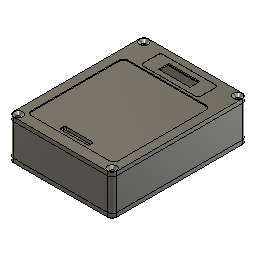
WiegandEmulator (Autodesk Fusion 360 design; units mm, degrees)
Autodesk Fusion 360 part; units mm, degrees
sketch "Sketch1" plane through (0, 0, 0) normal (0, 1, 0) x (1, 0, 0) in component "Core"
  line L0 (41.275, -53.975) -> (-41.275, -53.975)
  line L1 (-41.275, -53.975) -> (-41.275, 53.975)
  line L2 (-41.275, 53.975) -> (41.275, 53.975)
  line L3 (41.275, 53.975) -> (41.275, -53.975)
  line L4 (41.275, -53.975) -> (-41.275, 53.975) construction
  line L5 (-41.275, -53.975) -> (41.275, 53.975) construction
  dimension "d1" = 82.55
  dimension "d2" = 107.95
  constraint perpendicular L0 L1
  constraint parallel L0 L2
  constraint parallel L1 L3
  constraint horizontal L0
  constraint coincident L4 origin
  constraint coincident L5 origin
  measures "d1" distance of L1.end L2.end
  measures "d2" distance of L0.end L1.end
extrude "Extrude1" add sketch "Sketch1" along normal blind 25.4 makes body 1 in component "Core"
fillet "Fillet1" radius 3.81 4 edges at (41.275, 12.7, 53.975) (-41.275, 12.7, 53.975) (-41.275, 12.7, -53.975) (41.275, 12.7, -53.975) on bodies 1 in component "Core"
sketch "Sketch2" plane through (0, 25.4, 0) normal (0, 1, 0) x (-1, 0, 0) in component "Core"
  line L0 (-37.465, -53.975) -> (37.465, -53.975)
  line L1 (41.275, -50.165) -> (41.275, 50.165)
  line L2 (37.465, 53.975) -> (-37.465, 53.975)
  line L3 (-41.275, 50.165) -> (-41.275, -50.165)
  arc A0 (-41.275, -50.165) -> (-37.465, -53.975) centre (-37.465, -50.165) ccw
  arc A1 (37.465, -53.975) -> (41.275, -50.165) centre (37.465, -50.165) ccw
  arc A2 (41.275, 50.165) -> (37.465, 53.975) centre (37.465, 50.165) ccw
  arc A3 (-37.465, 53.975) -> (-41.275, 50.165) centre (-37.465, 50.165) ccw
  circle A4 centre (-37.465, 50.165) radius 1.8542
  circle A5 centre (37.465, 50.165) radius 1.8542
  circle A6 centre (37.465, -50.165) radius 1.8542
  circle A7 centre (-37.465, -50.165) radius 1.8542
  line L4 (38.735, -58.42) -> (38.735, 58.42) construction
  line L5 (-38.735, -46.5729) -> (-38.735, 46.5729)
  line L6 (-33.8729, 51.435) -> (33.8729, 51.435)
  line L7 (38.735, 46.5729) -> (38.735, -46.5729)
  arc A8 (41.0571, -51.435) -> (41.275, -50.165) centre (37.465, -50.165) ccw
  arc A9 (38.735, -46.5729) -> (33.8729, -51.435) centre (37.465, -50.165) ccw
  line L8 (33.8729, -51.435) -> (-33.8729, -51.435)
  line L9 (-38.735, -51.435) -> (-38.735, -51.516) construction
  arc A10 (-33.8729, -51.435) -> (-38.735, -46.5729) centre (-37.465, -50.165) ccw
  line L10 (-43.18, -51.435) -> (-41.0571, -51.435) construction
  line L11 (-38.816, -51.435) -> (-38.735, -51.435) construction
  line L12 (-33.8729, -51.435) -> (43.18, -51.435) construction
  arc A11 (33.8729, 51.435) -> (38.735, 46.5729) centre (37.465, 50.165) ccw
  arc A12 (-38.735, 46.5729) -> (-33.8729, 51.435) centre (-37.465, 50.165) ccw
  line L13 (-38.735, 51.516) -> (-38.735, 51.435) construction
  line L14 (-38.735, 46.5729) -> (-38.735, -46.5729) construction
  line L15 (43.18, 51.435) -> (-33.8729, 51.435) construction
  line L16 (-38.735, 51.435) -> (-38.816, 51.435) construction
  dimension "d10" = 3.7084
  dimension "d11" = 3.7084
  dimension "d12" = 3.7084
  dimension "d13" = 3.7084
  dimension "d14" = 2.54
  dimension "d15" = 2.54
  dimension "d16" = 2.54
  dimension "d17" = 2.54
  dimension "d18" = 3.81
  dimension "d19" = 3.81
  dimension "d21" = 3.81
  dimension "d22" = 3.81
  constraint concentric A3 A4
  constraint concentric A2 A5
  constraint concentric A1 A6
  constraint concentric A0 A7
  constraint perpendicular L0 L4
  constraint perpendicular L4 L15
  constraint perpendicular L13 L15
  constraint perpendicular L1 L10
  constraint concentric A1 A9
  constraint concentric A0 A10
  constraint coincident L5.end L13
  constraint coincident L6.end L15
  constraint coincident L4 L7.start
  constraint coincident L4 L7.end
  constraint coincident A8.start L10
  constraint concentric A8 A9
  constraint coincident A9.end L10
  constraint coincident L8.end L10
  constraint coincident A7 L9.end
  constraint coincident L9.start L10
  constraint collinear L9 L13
  constraint coincident A0 L10.end
  constraint coincident A7 L11.start
  constraint collinear L10 L11
  constraint collinear L11 L12
  constraint coincident A4 L13.start
  constraint collinear L13 L14
  constraint coincident L13.end L15
  constraint collinear L15 L16
  constraint coincident A4 L16.end
  constraint horizontal A2.centre A3.centre
  constraint vertical A1.centre A2.centre
  constraint vertical A0.centre A3.centre
  measures "d10" diameter of A4
  measures "d11" diameter of A5
  measures "d12" diameter of A6
  measures "d13" diameter of A7
  measures "d14" distance of L0 L10
  measures "d15" distance of L3 L13
  measures "d16" distance of L2 L15
  measures "d17" distance of L1 L4
  measures "d18" radius of A10
  measures "d19" radius of A9
  measures "d21" radius of A11
  measures "d22" radius of A12
extrude "Extrude2" cut sketch "Sketch2" against normal through all contours A4 | A5 | A6 | A7 | L5 L6 L7 A9 L8 A10 A11 A12 bodies 1 in component "Core"
sketch "Sketch1 (2)" plane through (0, 25.4, 0) normal (0, 1, 0) x (-1, 0, 0) in component "TopLid"
  circle A0 centre (-37.465, 50.165) radius 1.8542
  circle A1 centre (37.465, 50.165) radius 1.8542
  circle A2 centre (37.465, -50.165) radius 1.8542
  arc A3 (33.8729, 51.435) -> (38.735, 46.5729) centre (37.465, 50.165) ccw
  line L0 (38.735, 46.5729) -> (38.735, -46.5729)
  arc A4 (38.735, -46.5729) -> (33.8729, -51.435) centre (37.465, -50.165) ccw
  line L1 (33.8729, -51.435) -> (-33.8729, -51.435)
  arc A5 (-33.8729, -51.435) -> (-38.735, -46.5729) centre (-37.465, -50.165) ccw
  line L2 (-38.735, -46.5729) -> (-38.735, 46.5729)
  arc A6 (-38.735, 46.5729) -> (-33.8729, 51.435) centre (-37.465, 50.165) ccw
  line L3 (-33.8729, 51.435) -> (33.8729, 51.435)
  circle A7 centre (-37.465, -50.165) radius 1.8542
  arc A8 (-41.275, -50.165) -> (-37.465, -53.975) centre (-37.465, -50.165) ccw
  line L4 (-37.465, -53.975) -> (37.465, -53.975)
  arc A9 (37.465, -53.975) -> (41.275, -50.165) centre (37.465, -50.165) ccw
  line L5 (41.275, -50.165) -> (41.275, 50.165)
  arc A10 (41.275, 50.165) -> (37.465, 53.975) centre (37.465, 50.165) ccw
  line L6 (37.465, 53.975) -> (-37.465, 53.975)
  arc A11 (-37.465, 53.975) -> (-41.275, 50.165) centre (-37.465, 50.165) ccw
  line L7 (-41.275, 50.165) -> (-41.275, -50.165)
  line L8 (41.275, -50.165) -> (41.275, 50.165)
  arc A12 (41.275, 50.165) -> (37.465, 53.975) centre (37.465, 50.165) ccw
  line L9 (37.465, 53.975) -> (-37.465, 53.975)
  arc A13 (-37.465, 53.975) -> (-41.275, 50.165) centre (-37.465, 50.165) ccw
  line L10 (-41.275, 50.165) -> (-41.275, -50.165)
  arc A14 (-41.275, -50.165) -> (-37.465, -53.975) centre (-37.465, -50.165) ccw
  line L11 (-37.465, -53.975) -> (37.465, -53.975)
  arc A15 (37.465, -53.975) -> (41.275, -50.165) centre (37.465, -50.165) ccw
  circle A16 centre (37.465, -50.165) radius 1.8542
  circle A17 centre (37.465, 50.165) radius 1.8542
  circle A18 centre (-37.465, 50.165) radius 1.8542
  circle A19 centre (-37.465, -50.165) radius 1.8542
  circle A20 centre (-37.465, 50.165) radius 1.524
  circle A21 centre (37.465, 50.165) radius 1.524
  circle A22 centre (37.465, -50.165) radius 1.524
  circle A23 centre (-37.465, -50.165) radius 1.524
  dimension "d26" = 3.048
  dimension "d27" = 3.048
  dimension "d28" = 3.048
  dimension "d29" = 3.048
  constraint concentric A18 A20
  constraint concentric A12 A21
  constraint concentric A16 A22
  constraint concentric A14 A23
  measures "d26" diameter of A20
  measures "d27" diameter of A21
  measures "d28" diameter of A22
  measures "d29" diameter of A23
extrude "Extrude1'" add sketch "Sketch1 (2)" along normal blind 3.175 separate body contours A0 A18 | A1 A17 | A2 A16 | A3 L0 A4 L1 A5 L2 A6 L3 | A7 A19 | A8 L4 A9 L5 A10 L6 A11 L7 L8 A12 L9 A13 L10 A14 L11 A15 | A20 | A21 | A22 | A23 makes body 2 in component "TopLid"
extrude "Extrude2'" cut sketch "Sketch1 (2)" along normal through all contours A20 | A21 | A22 | A23 bodies 2 in component "TopLid"
sketch "Sketch2 (2)" plane through (0, 28.575, 0) normal (0, 1, 0) x (-1, 0, 0) in component "TopLid"
  circle A0 centre (-37.465, 50.165) radius 1.524
  circle A1 centre (-37.465, -50.165) radius 1.524
  circle A2 centre (37.465, 50.165) radius 1.524
  circle A3 centre (37.465, -50.165) radius 1.524
  arc A4 (37.465, -53.975) -> (41.275, -50.165) centre (37.465, -50.165) ccw
  line L0 (41.275, -50.165) -> (41.275, 50.165)
  arc A5 (41.275, 50.165) -> (37.465, 53.975) centre (37.465, 50.165) ccw
  line L1 (37.465, 53.975) -> (-37.465, 53.975)
  arc A6 (-37.465, 53.975) -> (-41.275, 50.165) centre (-37.465, 50.165) ccw
  line L2 (-41.275, 50.165) -> (-41.275, -50.165)
  arc A7 (-41.275, -50.165) -> (-37.465, -53.975) centre (-37.465, -50.165) ccw
  line L3 (-37.465, -53.975) -> (37.465, -53.975)
  line L4 (31.171, 45.975) -> (-31.171, 45.975)
  line L5 (-34.671, 42.475) -> (-34.671, -27.525)
  line L6 (-31.171, -31.025) -> (31.171, -31.025)
  line L7 (34.671, -27.525) -> (34.671, 42.475)
  arc A8 (34.671, 42.475) -> (31.171, 45.975) centre (31.171, 42.475) ccw
  arc A9 (-34.671, -27.525) -> (-31.171, -31.025) centre (-31.171, -27.525) ccw
  line L8 (34.671, -31.025) -> (-34.671, 45.975) construction
  arc A10 (31.171, -31.025) -> (34.671, -27.525) centre (31.171, -27.525) ccw
  arc A11 (-31.171, 45.975) -> (-34.671, 42.475) centre (-31.171, 42.475) ccw
  line L9 (-21, -49.025) -> (21, -49.025)
  line L10 (23, -47.025) -> (23, -35.025)
  line L11 (21, -33.025) -> (-21, -33.025)
  line L12 (-23, -35.025) -> (-23, -47.025)
  line L13 (-23, -49.025) -> (23, -33.025) construction
  line L14 (23, -49.025) -> (-23, -33.025) construction
  arc A12 (21, -49.025) -> (23, -47.025) centre (21, -47.025) ccw
  arc A13 (23, -35.025) -> (21, -33.025) centre (21, -35.025) ccw
  arc A14 (-21, -33.025) -> (-23, -35.025) centre (-21, -35.025) ccw
  arc A15 (-23, -47.025) -> (-21, -49.025) centre (-21, -47.025) ccw
  point P0 (34.671, 45.975)
  point P1 (0, -41.025)
  dimension "d31" = 69.342
  dimension "d32" = 77
  dimension "d33" = 34.671
  dimension "d34" = 8
  dimension "d35" = 3.5
  dimension "d36" = 3.5
  dimension "d37" = 3.5
  dimension "d38" = 3.5
  dimension "d50" = 46
  dimension "d51" = 16
  dimension "d52" = 10
  dimension "d53" = 11.671
  dimension "d54" = 2
  dimension "d55" = 2
  dimension "d56" = 2
  dimension "d57" = 2
  constraint horizontal L4
  constraint vertical L5
  constraint horizontal L6
  constraint vertical L7
  constraint coincident P0 L7
  constraint coincident P0 L4
  constraint tangent L7 A8
  constraint tangent L4 A8
  constraint tangent L6 A9
  constraint tangent L5 A9
  constraint coincident L8.start L6
  constraint coincident L8.start L7
  constraint tangent L6 A10
  constraint tangent L7 A10
  constraint coincident L8.end L4
  constraint coincident L8.end L5
  constraint tangent L4 A11
  constraint tangent L5 A11
  constraint perpendicular L9 L10
  constraint parallel L9 L11
  constraint parallel L10 L12
  constraint horizontal L9
  constraint coincident L13 P1
  constraint coincident L14 P1
  constraint coincident L14.start L9
  constraint coincident L14.start L10
  constraint tangent L9 A12
  constraint tangent L10 A12
  constraint coincident L13.end L10
  constraint coincident L13.end L11
  constraint tangent L10 A13
  constraint tangent L11 A13
  constraint coincident L14.end L12
  constraint coincident L14.end L11
  constraint tangent L12 A14
  constraint tangent L11 A14
  constraint coincident L13.start L9
  constraint coincident L13.start L12
  constraint tangent L9 A15
  constraint tangent L12 A15
  measures "d31" distance of P0 L8.end
  measures "d32" distance of P0 L8.start
  measures "d33" distance of origin L7
  measures "d34" distance of L1 L4
  measures "d35" radius of A8
  measures "d36" radius of A9
  measures "d37" radius of A10
  measures "d38" radius of A11
  measures "d50" distance of L13.end L14.end
  measures "d51" distance of L14.start L13.end
  measures "d52" distance of L6 P1
  measures "d53" distance of L7 L10
  measures "d54" radius of A12
  measures "d55" radius of A13
  measures "d56" radius of A14
  measures "d57" radius of A15
extrude "Extrude3" cut sketch "Sketch2 (2)" against normal blind 0.75 contours L4 L5 L6 L7 A8 A9 A10 A11 bodies 2 in component "TopLid"
sketch "Sketch3" plane through (0, 27.825, 0) normal (0, 1, 0) x (-1, 0, 0) in component "TopLid"
  arc A0 (-31.171, 45.975) -> (-34.671, 42.475) centre (-31.171, 42.475) ccw
  line L0 (-34.671, 42.475) -> (-34.671, -27.525)
  arc A1 (-34.671, -27.525) -> (-31.171, -31.025) centre (-31.171, -27.525) ccw
  line L1 (-31.171, -31.025) -> (31.171, -31.025)
  arc A2 (31.171, -31.025) -> (34.671, -27.525) centre (31.171, -27.525) ccw
  line L2 (34.671, -27.525) -> (34.671, 42.475)
  arc A3 (34.671, 42.475) -> (31.171, 45.975) centre (31.171, 42.475) ccw
  line L3 (31.171, 45.975) -> (-31.171, 45.975)
  line L4 (10.5, 42.975) -> (-10.5, 42.975)
  line L5 (-11.5, 41.975) -> (-11.5, 39.975)
  line L6 (-10.5, 38.975) -> (10.5, 38.975)
  line L7 (11.5, 39.975) -> (11.5, 41.975)
  arc A4 (11.5, 41.975) -> (10.5, 42.975) centre (10.5, 41.975) ccw
  arc A5 (10.5, 38.975) -> (11.5, 39.975) centre (10.5, 39.975) ccw
  arc A6 (-10.5, 42.975) -> (-11.5, 41.975) centre (-10.5, 41.975) ccw
  arc A7 (-11.5, 39.975) -> (-10.5, 38.975) centre (-10.5, 39.975) ccw
  point P0 (11.5, 42.975)
  point P1 (-11.5, 42.975)
  point P2 (11.5, 38.975)
  dimension "d41" = 23
  dimension "d42" = 4
  dimension "d43" = 11.5
  dimension "d44" = 7
  dimension "d45" = 1
  dimension "d46" = 1
  dimension "d47" = 1
  dimension "d48" = 1
  constraint horizontal L4
  constraint vertical L5
  constraint horizontal L6
  constraint vertical L7
  constraint coincident P0 L4
  constraint coincident P0 L7
  constraint tangent L4 A4
  constraint tangent L7 A4
  constraint coincident P2 L6
  constraint coincident P2 L7
  constraint tangent L6 A5
  constraint tangent L7 A5
  constraint coincident P1 L4
  constraint coincident P1 L5
  constraint tangent L4 A6
  constraint tangent L5 A6
  constraint tangent L5 A7
  constraint tangent L6 A7
  measures "d41" distance of P0 P1
  measures "d42" distance of P0 P2
  measures "d43" distance of origin L5
  measures "d44" distance of L3 L6
  measures "d45" radius of A4
  measures "d46" radius of A5
  measures "d47" radius of A6
  measures "d48" radius of A7
extrude "Extrude4" cut sketch "Sketch3" against normal through all contours L4 L5 L6 L7 A4 A5 A6 A7 bodies 2 in component "TopLid"
extrude "Extrude5" cut sketch "Sketch2 (2)" against normal through all contours L9 L10 L11 L12 A12 A13 A14 A15 bodies 2 in component "TopLid"
chamfer "Chamfer2" distance 2 angle 45 4 edges at (-36.0441, 28.575, 50.7161) (38.8859, 28.575, 50.7161) (-36.0441, 28.575, -49.6139) (38.8859, 28.575, -49.6139) on bodies 2 in component "TopLid"
sketch "Sketch1 (3)" plane through (0, 0, 0) normal (0, -1, 0) x (1, 0, 0) in component "BottomLid"
  circle A0 centre (37.465, 50.165) radius 1.8542
  circle A1 centre (-37.465, 50.165) radius 1.8542
  circle A2 centre (-37.465, -50.165) radius 1.8542
  arc A3 (-38.735, 46.5729) -> (-33.8729, 51.435) centre (-37.465, 50.165) ccw
  line L0 (-33.8729, 51.435) -> (33.8729, 51.435)
  arc A4 (33.8729, 51.435) -> (38.735, 46.5729) centre (37.465, 50.165) ccw
  line L1 (38.735, 46.5729) -> (38.735, -46.5729)
  arc A5 (38.735, -46.5729) -> (33.8729, -51.435) centre (37.465, -50.165) ccw
  line L2 (33.8729, -51.435) -> (-33.8729, -51.435)
  arc A6 (-33.8729, -51.435) -> (-38.735, -46.5729) centre (-37.465, -50.165) ccw
  line L3 (-38.735, -46.5729) -> (-38.735, 46.5729)
  circle A7 centre (37.465, -50.165) radius 1.8542
  arc A8 (37.465, -53.975) -> (41.275, -50.165) centre (37.465, -50.165) ccw
  line L4 (41.275, -50.165) -> (41.275, 50.165)
  arc A9 (41.275, 50.165) -> (37.465, 53.975) centre (37.465, 50.165) ccw
  line L5 (37.465, 53.975) -> (-37.465, 53.975)
  arc A10 (-37.465, 53.975) -> (-41.275, 50.165) centre (-37.465, 50.165) ccw
  line L6 (-41.275, 50.165) -> (-41.275, -50.165)
  arc A11 (-41.275, -50.165) -> (-37.465, -53.975) centre (-37.465, -50.165) ccw
  line L7 (-37.465, -53.975) -> (37.465, -53.975)
  line L8 (-41.275, 50.165) -> (-41.275, -50.165)
  arc A12 (-37.465, 53.975) -> (-41.275, 50.165) centre (-37.465, 50.165) ccw
  line L9 (37.465, 53.975) -> (-37.465, 53.975)
  arc A13 (41.275, 50.165) -> (37.465, 53.975) centre (37.465, 50.165) ccw
  line L10 (41.275, -50.165) -> (41.275, 50.165)
  arc A14 (37.465, -53.975) -> (41.275, -50.165) centre (37.465, -50.165) ccw
  line L11 (-37.465, -53.975) -> (37.465, -53.975)
  arc A15 (-41.275, -50.165) -> (-37.465, -53.975) centre (-37.465, -50.165) ccw
  circle A16 centre (-37.465, 50.165) radius 1.8542
  circle A17 centre (37.465, 50.165) radius 1.8542
  circle A18 centre (37.465, -50.165) radius 1.8542
  circle A19 centre (-37.465, -50.165) radius 1.8542
extrude "Extrude1''" add sketch "Sketch1 (3)" along normal blind 3.175 separate body contours A3 L0 A4 L1 A5 L2 A6 L3 | A8 L4 A9 L5 A10 L6 A11 L7 L8 A12 L9 A13 L10 A14 L11 A15 makes body 3 in component "BottomLid"
chamfer "Chamfer1" distance 1.75 angle 45 4 edges at (35.7363, -3.175, 50.8355) (-39.1937, -3.175, 50.8355) (-39.1937, -3.175, -49.4945) (35.7363, -3.175, -49.4945) on bodies 3 in component "BottomLid"
sketch "Sketch2 (3)" plane through (0, 0, 0) normal (0, 1, 0) x (-1, 0, 0) in component "BottomLid"
  circle A0 centre (-37.465, 50.165) radius 1.8542
  circle A1 centre (-37.465, -50.165) radius 1.8542
  circle A2 centre (37.465, -50.165) radius 1.8542
  circle A3 centre (37.465, 50.165) radius 1.8542
  arc A4 (37.465, -53.975) -> (41.275, -50.165) centre (37.465, -50.165) ccw
  line L0 (41.275, -50.165) -> (41.275, 50.165)
  arc A5 (41.275, 50.165) -> (37.465, 53.975) centre (37.465, 50.165) ccw
  line L1 (37.465, 53.975) -> (-37.465, 53.975)
  arc A6 (-37.465, 53.975) -> (-41.275, 50.165) centre (-37.465, 50.165) ccw
  line L2 (-41.275, 50.165) -> (-41.275, -50.165)
  arc A7 (-41.275, -50.165) -> (-37.465, -53.975) centre (-37.465, -50.165) ccw
  line L3 (-37.465, -53.975) -> (37.465, -53.975)
  circle A8 centre (0, -38.975) radius 6.1
  circle A9 centre (0, 38.975) radius 6.1
  dimension "d64" = 12.2
  dimension "d65" = 12.2
  dimension "d66" = 15
  dimension "d67" = 15
  dimension "d68" = 41.275
  constraint vertical A8.centre A9.centre
  measures "d64" diameter of A8
  measures "d65" diameter of A9
  measures "d66" distance of L1 A9.centre
  measures "d67" distance of L3 A8.centre
  measures "d68" distance of L2 A8.centre
extrude "Extrude2''" cut sketch "Sketch2 (3)" against normal blind 2.54 contours A8 | A9 bodies 3 in component "BottomLid"
fillet "Fillet1'" radius 0.5 2 edges at (5.6872, 0, 41.1809) (5.6872, 0, -36.7691) on bodies 3 in component "BottomLid"
ref_plane "WorkPlane1" through (0, 25.4, 0) normal (0, -1, 0) x (1, 0, 0) in component "DisplayInsert"
sketch "Sketch1 (4)" plane through (0, 25.4, 0) normal (0, -1, 0) x (1, 0, 0) in component "DisplayInsert"
  line L0 (-21, -49.025) -> (21, -49.025)
  arc A0 (21, -49.025) -> (23, -47.025) centre (21, -47.025) ccw
  line L1 (23, -47.025) -> (23, -35.025)
  arc A1 (23, -35.025) -> (21, -33.025) centre (21, -35.025) ccw
  line L2 (21, -33.025) -> (-21, -33.025)
  arc A2 (-21, -33.025) -> (-23, -35.025) centre (-21, -35.025) ccw
  line L3 (-23, -35.025) -> (-23, -47.025)
  arc A3 (-23, -47.025) -> (-21, -49.025) centre (-21, -47.025) ccw
  line L4 (23.5, -47.025) -> (23.5, -35.025)
  arc A4 (23.5, -35.025) -> (21, -32.525) centre (21, -35.025) ccw
  line L5 (21, -32.525) -> (-21, -32.525)
  arc A5 (-21, -32.525) -> (-23.5, -35.025) centre (-21, -35.025) ccw
  line L6 (-23.5, -35.025) -> (-23.5, -47.025)
  arc A6 (-23.5, -47.025) -> (-21, -49.525) centre (-21, -47.025) ccw
  line L7 (-21, -49.525) -> (21, -49.525)
  arc A7 (21, -49.525) -> (23.5, -47.025) centre (21, -47.025) ccw
  line L8 (22.9, -47.025) -> (22.9, -35.025)
  arc A8 (22.9, -35.025) -> (21, -33.125) centre (21, -35.025) ccw
  line L9 (21, -33.125) -> (-21, -33.125)
  arc A9 (-21, -33.125) -> (-22.9, -35.025) centre (-21, -35.025) ccw
  line L10 (-22.9, -35.025) -> (-22.9, -47.025)
  arc A10 (-22.9, -47.025) -> (-21, -48.925) centre (-21, -47.025) ccw
  line L11 (-21, -48.925) -> (21, -48.925)
  arc A11 (21, -48.925) -> (22.9, -47.025) centre (21, -47.025) ccw
  dimension "d73" = 0.5
  dimension "d89" = -0.1
extrude "Extrude1'''" add sketch "Sketch1 (4)" against normal blind 3.175 separate body contours L8 A8 L9 A9 L10 A10 L11 A11 makes body 4 in component "DisplayInsert"
extrude "Extrude2'''" add sketch "Sketch1 (4)" along normal blind 1 contours L0 A0 L1 A1 L2 A2 L3 A3 | L4 A4 L5 A5 L6 A6 L7 A7 | L8 A8 L9 A9 L10 A10 L11 A11 bodies 4 in component "DisplayInsert"
sketch "Sketch2 (4)" plane through (0, 28.575, 0) normal (0, 1, 0) x (-1, 0, 0) in component "DisplayInsert"
  line L0 (-12.5, -37.025) -> (12.5, -37.025)
  line L1 (12.5, -37.025) -> (12.5, -45.025)
  line L2 (12.5, -45.025) -> (-12.5, -45.025)
  line L3 (-12.5, -45.025) -> (-12.5, -37.025)
  line L4 (-12.5, -37.025) -> (12.5, -45.025) construction
  line L5 (12.5, -37.025) -> (-12.5, -45.025) construction
  arc A0 (-22.9, -47.025) -> (-21, -48.925) centre (-21, -47.025) ccw
  line L6 (-21, -48.925) -> (21, -48.925)
  arc A1 (21, -48.925) -> (22.9, -47.025) centre (21, -47.025) ccw
  line L7 (22.9, -47.025) -> (22.9, -35.025)
  arc A2 (22.9, -35.025) -> (21, -33.125) centre (21, -35.025) ccw
  line L8 (21, -33.125) -> (-21, -33.125)
  arc A3 (-21, -33.125) -> (-22.9, -35.025) centre (-21, -35.025) ccw
  line L9 (-22.9, -35.025) -> (-22.9, -47.025)
  point P0 (0, -41.025)
  dimension "d78" = 25
  dimension "d79" = 8
  dimension "d90" = 10.4
  dimension "d91" = 3.9
  constraint perpendicular L0 L1
  constraint parallel L0 L2
  constraint parallel L1 L3
  constraint horizontal L0
  constraint coincident L4 P0
  constraint coincident L5 P0
  measures "d78" distance of L1.end L2.end
  measures "d79" distance of L0.end L1.end
  measures "d90" distance of L3 L9
  measures "d91" distance of L2 L6
extrude "Extrude3'" cut sketch "Sketch2 (4)" against normal through all contours L0 L1 L2 L3 bodies 4 in component "DisplayInsert"
sketch "Sketch3 (2)" plane through (0, 24.4, 0) normal (0, -1, 0) x (1, 0, 0) in component "DisplayInsert"
  line L0 (12.5, -37.025) -> (12.5, -45.025)
  line L1 (12.5, -45.025) -> (-12.5, -45.025)
  line L2 (-12.5, -45.025) -> (-12.5, -37.025)
  line L3 (-12.5, -37.025) -> (12.5, -37.025)
  arc A0 (21, -49.525) -> (23.5, -47.025) centre (21, -47.025) ccw
  line L4 (23.5, -47.025) -> (23.5, -35.025)
  arc A1 (23.5, -35.025) -> (21, -32.525) centre (21, -35.025) ccw
  line L5 (21, -32.525) -> (-21, -32.525)
  arc A2 (-21, -32.525) -> (-23.5, -35.025) centre (-21, -35.025) ccw
  line L6 (-23.5, -35.025) -> (-23.5, -47.025)
  arc A3 (-23.5, -47.025) -> (-21, -49.525) centre (-21, -47.025) ccw
  line L7 (-21, -49.525) -> (21, -49.525)
  line L8 (18.75, -47.525) -> (-19.75, -47.525)
  line L9 (-19.75, -47.525) -> (-19.75, -34.525)
  line L10 (-19.75, -34.525) -> (18.75, -34.525)
  line L11 (18.75, -34.525) -> (18.75, -47.525)
  line L12 (18.75, -47.525) -> (-19.75, -34.525) construction
  line L13 (-19.75, -47.525) -> (18.75, -34.525) construction
  point P0 (-0.5, -41.025)
  dimension "d83" = 38.5
  dimension "d84" = 13
  dimension "d85" = 7.25
  dimension "d86" = 2.5
  constraint perpendicular L8 L9
  constraint parallel L8 L10
  constraint parallel L9 L11
  constraint horizontal L8
  constraint coincident L12 P0
  constraint coincident L13 P0
  measures "d83" distance of L9.end L10.end
  measures "d84" distance of L8.end L9.end
  measures "d85" distance of L2 L9
  measures "d86" distance of L3 L10
extrude "Extrude4'" cut sketch "Sketch3 (2)" against normal blind 3.2 contours L8 L9 L10 L11 bodies 4 in component "DisplayInsert"
sketch "Sketch1 (5)" plane through (0, 25.4, 0) normal (0, -1, 0) x (1, 0, 0) in component "ArduinoHolder"
  line L0 (-21, -33.025) -> (21, -33.025)
  arc A0 (23, -35.025) -> (21, -33.025) centre (21, -35.025) ccw
  line L1 (23, -35.025) -> (23, -47.025)
  arc A1 (21, -49.025) -> (23, -47.025) centre (21, -47.025) ccw
  line L2 (21, -49.025) -> (-21, -49.025)
  arc A2 (-23, -47.025) -> (-21, -49.025) centre (-21, -47.025) ccw
  line L3 (-23, -47.025) -> (-23, -35.025)
  arc A3 (-21, -33.025) -> (-23, -35.025) centre (-21, -35.025) ccw
  line L4 (-10.5, 42.975) -> (10.5, 42.975)
  arc A4 (11.5, 41.975) -> (10.5, 42.975) centre (10.5, 41.975) ccw
  line L5 (11.5, 41.975) -> (11.5, 39.975)
  arc A5 (10.5, 38.975) -> (11.5, 39.975) centre (10.5, 39.975) ccw
  line L6 (10.5, 38.975) -> (-10.5, 38.975)
  arc A6 (-11.5, 39.975) -> (-10.5, 38.975) centre (-10.5, 39.975) ccw
  line L7 (-11.5, 39.975) -> (-11.5, 41.975)
  arc A7 (-10.5, 42.975) -> (-11.5, 41.975) centre (-10.5, 41.975) ccw
  circle A8 centre (37.465, 50.165) radius 1.524
  circle A9 centre (37.465, -50.165) radius 1.524
  circle A10 centre (-37.465, 50.165) radius 1.524
  circle A11 centre (-37.465, -50.165) radius 1.524
  arc A12 (-41.275, -50.165) -> (-37.465, -53.975) centre (-37.465, -50.165) ccw
  line L8 (-37.465, -53.975) -> (37.465, -53.975)
  arc A13 (37.465, -53.975) -> (41.275, -50.165) centre (37.465, -50.165) ccw
  line L9 (41.275, -50.165) -> (41.275, 50.165)
  arc A14 (41.275, 50.165) -> (37.465, 53.975) centre (37.465, 50.165) ccw
  line L10 (37.465, 53.975) -> (-37.465, 53.975)
  arc A15 (-37.465, 53.975) -> (-41.275, 50.165) centre (-37.465, 50.165) ccw
  line L11 (-41.275, 50.165) -> (-41.275, -50.165)
  line L12 (-38.7, 15) -> (38.7, 15)
  line L13 (38.7, 15) -> (38.7, 0)
  line L14 (38.7, 0) -> (-38.7, 0)
  line L15 (-38.7, 0) -> (-38.7, 15)
  dimension "d92" = 77.4
  dimension "d93" = 15
  dimension "d94" = 38.7
  constraint horizontal L12
  constraint vertical L13
  constraint horizontal L14
  constraint vertical L15
  constraint coincident origin L14
  measures "d92" distance of L12.start L12.end
  measures "d93" distance of L12.start L14.end
  measures "d94" distance of origin L13
extrude "Extrude1''''" add sketch "Sketch1 (5)" along normal blind 20 separate body contours L12 L13 L14 L15 makes body 5 in component "ArduinoHolder"
sketch "Sketch2 (5)" plane through (0, 0, 0) normal (0, 0, -1) x (-1, 0, 0) in component "ArduinoHolder"
  line L0 (38.7, 25.4) -> (-38.7, 25.4)
  line L1 (-38.7, 25.4) -> (-38.7, 5.4)
  line L2 (-38.7, 5.4) -> (38.7, 5.4)
  line L3 (38.7, 5.4) -> (38.7, 25.4)
  line L4 (35, 25.4) -> (-35, 25.4)
  line L5 (-35, 25.4) -> (-35, 5.4)
  line L6 (-35, 5.4) -> (35, 5.4)
  line L7 (35, 5.4) -> (35, 25.4)
  point P0 (0, 5.4)
  point P1 (0, 5.4)
  dimension "d97" = 20
  dimension "d98" = 70
  constraint horizontal L4
  constraint vertical L5
  constraint horizontal L6
  constraint vertical L7
  constraint coincident L0 L4.start
  constraint midpoint L6 P1
  constraint midpoint L2 P1
  constraint coincident P1 P0
  measures "d97" distance of L4.start L6.end
  measures "d98" distance of L4.start L4.end
extrude "Extrude2''''" cut sketch "Sketch2 (5)" against normal blind 10 contours L0 L2 L4 L5 L6 L7 bodies 5 in component "ArduinoHolder"
fillet "Fillet1''" radius 1 4 edges at (-38.7, 25.4, 7.5) (38.7, 25.4, 7.5) (38.7, 5.4, 7.5) (-38.7, 5.4, 7.5) on bodies 5 in component "ArduinoHolder"
sketch "Sketch5" plane through (0, 0, 10) normal (0, 0, -1) x (-1, 0, 0) in component "ArduinoHolder"
  line L0 (35, 5.4) -> (35, 25.4)
  line L1 (35, 25.4) -> (-35, 25.4)
  line L2 (-35, 25.4) -> (-35, 5.4)
  line L3 (-35, 5.4) -> (35, 5.4)
  line L4 (-33, 25.4) -> (10.5, 25.4)
  line L5 (10.5, 25.4) -> (10.5, 7.15)
  line L6 (10.5, 7.15) -> (-33, 7.15)
  line L7 (-33, 7.15) -> (-33, 25.4)
  dimension "d113" = 43.5
  dimension "d114" = 18.25
  dimension "d115" = 2
  constraint horizontal L4
  constraint vertical L5
  constraint horizontal L6
  constraint vertical L7
  constraint coincident L1 L4.start
  measures "d113" distance of L4.start L4.end
  measures "d114" distance of L4.start L6.end
  measures "d115" distance of L2 L7
extrude "Extrude5'" cut sketch "Sketch5" against normal blind 2.1 contours L1 L4 L5 L6 L7 bodies 5 in component "ArduinoHolder"
sketch "Sketch7" plane through (0, 0, 12.1) normal (0, 0, -1) x (-1, 0, 0) in component "ArduinoHolder"
  line L0 (-33, 7.15) -> (10.5, 7.15)
  line L1 (10.5, 7.15) -> (10.5, 25.4)
  line L2 (10.5, 25.4) -> (-33, 25.4)
  line L3 (-33, 25.4) -> (-33, 7.15)
  line L4 (-30.75, 25.4) -> (8.25, 25.4)
  line L5 (8.25, 25.4) -> (8.25, 21.4)
  line L6 (8.25, 21.4) -> (-30.75, 21.4)
  line L7 (-30.75, 21.4) -> (-30.75, 25.4)
  line L8 (-30.75, 7.15) -> (8.25, 7.15)
  line L9 (8.25, 7.15) -> (8.25, 11.15)
  line L10 (8.25, 11.15) -> (-30.75, 11.15)
  line L11 (-30.75, 11.15) -> (-30.75, 7.15)
  dimension "d123" = 39
  dimension "d124" = 4
  dimension "d125" = 2.25
  dimension "d126" = 4
  dimension "d127" = 39
  dimension "d128" = 2.25
  constraint horizontal L4
  constraint vertical L5
  constraint horizontal L6
  constraint vertical L7
  constraint coincident L2 L4.start
  constraint horizontal L8
  constraint vertical L9
  constraint horizontal L10
  constraint vertical L11
  constraint coincident L0 L8.start
  measures "d123" distance of L4.start L4.end
  measures "d124" distance of L4.start L6.end
  measures "d125" distance of L3 L7
  measures "d126" distance of L8.start L10.end
  measures "d127" distance of L8.start L8.end
  measures "d128" distance of L3 L11
extrude "Extrude7" cut sketch "Sketch7" against normal through all contours L0 L8 L9 L10 L11 | L2 L4 L5 L6 L7 bodies 5 in component "ArduinoHolder"
sketch "Sketch8" plane through (0, 0, 12.1) normal (0, 0, -1) x (-1, 0, 0) in component "ArduinoHolder"
  line L0 (8.25, 25.4) -> (8.25, 21.4)
  line L1 (8.25, 21.4) -> (-30.75, 21.4)
  line L2 (-30.75, 21.4) -> (-30.75, 25.4)
  line L3 (-30.75, 25.4) -> (-33, 25.4)
  line L4 (-33, 25.4) -> (-33, 7.15)
  line L5 (-33, 7.15) -> (-30.75, 7.15)
  line L6 (-30.75, 7.15) -> (-30.75, 11.15)
  line L7 (-30.75, 11.15) -> (8.25, 11.15)
  line L8 (8.25, 11.15) -> (8.25, 7.15)
  line L9 (8.25, 7.15) -> (10.5, 7.15)
  line L10 (10.5, 7.15) -> (10.5, 25.4)
  line L11 (10.5, 25.4) -> (8.25, 25.4)
  line L12 (-33, 21.4) -> (10.5, 21.4)
  line L13 (10.5, 21.4) -> (10.5, 11.15)
  line L14 (10.5, 11.15) -> (-33, 11.15)
  line L15 (-33, 11.15) -> (-33, 21.4)
  constraint horizontal L12
  constraint vertical L13
  constraint horizontal L14
  constraint vertical L15
  constraint coincident L10 L13.end
  constraint coincident L4 L12.start
extrude "Extrude8" cut sketch "Sketch8" against normal through all contours L1 L4 L7 L10 L12 L13 L14 L15 bodies 5 in component "ArduinoHolder"
fillet "Fillet4" radius 0.5 6 edges at (30.75, 25.4, 13.55) (30.75, 21.4, 13.55) (30.75, 11.15, 13.55) (-8.25, 21.4, 13.55) (-8.25, 25.4, 13.55) (-8.25, 11.15, 13.55) on bodies 5 in component "ArduinoHolder"
sketch "Sketch9" plane through (0, 0, 10) normal (0, 0, -1) x (-1, 0, 0) in component "ArduinoHolder"
  line L0 (-33, 7.15) -> (-33, 25.4)
  line L1 (-33, 25.4) -> (-35, 25.4)
  line L2 (-35, 25.4) -> (-35, 5.4)
  line L3 (-35, 5.4) -> (35, 5.4)
  line L4 (35, 5.4) -> (35, 25.4)
  line L5 (35, 25.4) -> (10.5, 25.4)
  line L6 (10.5, 25.4) -> (10.5, 7.15)
  line L7 (10.5, 7.15) -> (-33, 7.15)
  line L8 (10.5, 16.275) -> (35, 16.275) construction
  line L9 (10.5, 22.275) -> (30.5, 22.275)
  line L10 (30.5, 22.275) -> (30.5, 10.275)
  line L11 (30.5, 10.275) -> (10.5, 10.275)
  line L12 (10.5, 10.275) -> (10.5, 22.275)
  line L13 (12.5, 22.275) -> (12.5, 10.275)
  dimension "d132" = 20
  dimension "d133" = 12
  dimension "d134" = 6
  dimension "d138" = 2
  constraint midpoint L6 L8.start
  constraint coincident L4 L8.end
  constraint perpendicular L4 L8
  constraint horizontal L9
  constraint vertical L10
  constraint horizontal L11
  constraint vertical L12
  constraint coincident L6 L9.start
  constraint coincident L9 L13.start
  constraint coincident L11 L13.end
  constraint perpendicular L11 L13
  measures "d132" distance of L9.start L9.end
  measures "d133" distance of L9.start L11.end
  measures "d134" distance of L8 L11
  measures "d138" distance of L12 L13
extrude "Extrude9" cut sketch "Sketch9" against normal blind 2.5 contours L6 L9 L11 L12 L13 | L9 L10 L11 L13 bodies 5 in component "ArduinoHolder"
chamfer "Chamfer1'" distance 2.5 angle 45 1 edges at (-30.5, 16.275, 12.5) on bodies 5 in component "ArduinoHolder"
extrude "Extrude10" add sketch "Sketch9" against normal up to surface (2.5 mm away) contours L6 L9 L11 L12 L13 bodies 5 in component "ArduinoHolder"
component "Core" placed x (1, 0, 0) y (0, 1, 0) z (0, 0, 1) at (0, 0, 0)
component "TopLid" placed x (1, 0, 0) y (0, 1, 0) z (0, 0, 1) at (0, 0, 0)
component "BottomLid" placed x (1, 0, 0) y (0, 1, 0) z (0, 0, 1) at (0, 0, 0)
component "DisplayInsert" placed x (1, 0, 0) y (0, 1, 0) z (0, 0, 1) at (0, 0, 0)
component "ArduinoHolder" placed x (1, 0, 0) y (0, 1, 0) z (0, 0, 1) at (0, 0, 0)
equation "d33 = 2.73 in / 2"
equation "d94 = ( 77.4 / 2 ) * 1 mm"
